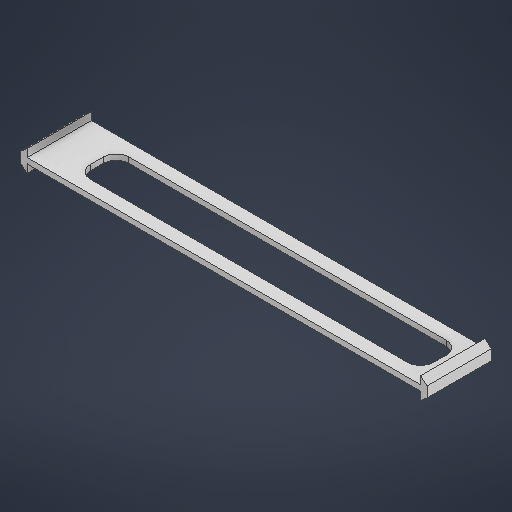
# Autodesk Inventor part: short slider
Saved by Autodesk Inventor 2026.2 (Build 302298000, 298)
## iProperties
Created: 2026-01-15
Part Number: short slider
Material: Generic
Document SubType Name: Modeling
Designer: dongr
Density: 1 g/cm^3
Appearance: Default
Author: dongr
Autodesk Inventor part; units mm, degrees
ref_plane "YZ Plane" through (0, 0, 0) normal (1, 0, 0) x (0, 1, 0)
ref_plane "XZ Plane" through (0, 0, 0) normal (0, 1, 0) x (-1, 0, 0)
ref_plane "XY Plane" through (0, 0, 0) normal (0, 0, 1) x (1, 0, 0)
sketch "Sketch1" plane through (0, 0, 0) normal (0, 1, 0) x (-1, 0, 0)
  line L0 (0, 0) -> (233.045, 0)
  line L1 (233.045, 0) -> (233.045, -38.1)
  line L2 (233.045, -38.1) -> (0, -38.1)
  line L3 (0, -38.1) -> (0, 0)
  dimension "d0" = 233.045
  dimension "d1" = 38.1
  constraints: 8 end point, 2 parallel, 1 horizontal, 1 perpendicular
  measures "d0" distance of L1.end L2.end
  measures "d1" distance of L0.end L1.end
extrude "Extrusion1" add sketch "Sketch1" along normal blind 3.2766
sketch "Sketch2" plane through (0, 3.2766, 0) normal (0, 1, 0) x (1, 0, 0)
  line L0 (-7.62, 7.62) -> (-210.82, 7.62)
  line L1 (-210.82, 7.62) -> (-210.82, 30.48)
  line L2 (-210.82, 30.48) -> (-7.62, 30.48)
  line L3 (-7.62, 30.48) -> (-7.62, 7.62)
  point P0 (0, 0)
  dimension "d4" = 203.2
  dimension "d5" = 22.86
  constraints: 8 end point, 2 parallel, 1 horizontal, 1 perpendicular
  measures "d4" distance of L1.end L2.end
  measures "d5" distance of L0.end L1.end
extrude "Extrusion2" cut sketch "Sketch2" against normal through all
fillet "Face Fillet1" radius 7.62 1 edges at (-210.82, 1.6383, -30.48)
fillet "Face Fillet2" radius 7.62 1 edges at (-210.82, 1.6383, -7.62)
fillet "Face Fillet3" radius 7.62 1 edges at (-7.62, 1.6383, -30.48)
fillet "Face Fillet4" radius 7.62 1 edges at (-7.62, 1.6383, -7.62)
sketch "Sketch3" plane through (-233.045, 0, 0) normal (0, 0, 1) x (1, 0, 0)
  line L0 (233.045, -4.826) -> (233.045, 7.8895)
  line L1 (233.045, 7.8895) -> (236.9365, 4.6242)
  line L2 (233.045, -4.826) -> (236.9365, -1.5606)
  line L3 (233.045, -4.826) -> (238.125, -4.826) construction
  line L4 (236.9365, -1.5606) -> (236.9365, 4.6242)
  line L5 (0, 7.8895) -> (0, -4.826)
  line L6 (0, -4.826) -> (-3.8915, -1.5606)
  line L7 (0, 7.8895) -> (-3.8915, 4.6242)
  line L8 (-3.8915, -1.5606) -> (-3.8915, 4.6242)
  point P0 (233.045, 0)
  dimension "d12" = 5.08
  dimension "d13" = 50
  dimension "d14" = 5.08
  dimension "d15" = 40
  dimension "d16" = 5.08
  dimension "d17" = 50
  dimension "d18" = 5.08
  constraints: 18 end point, 3 vertical, 1 equal length, 1 horizontal
  measures "d12" distance of L0.end L1.end
  measures "d13" angle of L0 L1
  measures "d14" distance of L0.start L2.end
  measures "d15" angle of L3 L2
  measures "d16" distance of L5.end L6.end
  measures "d17" angle of L5 L6
  measures "d18" distance of L5.start L7.end
extrude "Extrusion3" add sketch "Sketch3" against normal blind 38.1
body "Solid1"
